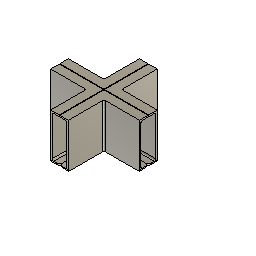
CornerProtectorForRatchetStraps (Autodesk Fusion 360 design; units mm, degrees)
Autodesk Fusion 360 part; units mm, degrees
sketch "Sketch1" plane through (0, 0, 0) normal (0, 0, 1) x (1, 0, 0)
  line L0 (0, 0) -> (0, 25)
  line L1 (0, 25) -> (1, 25)
  line L2 (1, 25) -> (1, 1)
  line L3 (1, 1) -> (25, 1)
  line L4 (25, 1) -> (25, 0)
  line L5 (25, 0) -> (0, 0)
  dimension "d1" = 1
  dimension "d2" = 25
  dimension "d3" = 25
  constraint coincident L0.start L5.end
  constraint vertical L0
  constraint perpendicular L0 L1
  constraint perpendicular L1 L2
  constraint perpendicular L2 L3
  constraint perpendicular L3 L4
  constraint horizontal L5
  constraint equal L1 L4
  measures "d1" distance of L0.end L1.end
  measures "d2" distance of L0.start L0.end
  measures "d3" distance of L4.end L0.start
extrude "Extrude2" add sketch "Sketch1" along normal blind 30
fillet "Fillet2" radius 1 2 edges at (1, 1, 15) (0, 0, 15)
ref_plane "WorkPlane1" through (12.5, 12.5, 15) normal (0, 0, 1) x (1, 0, 0)
sketch "Sketch3" plane through (0, 0, 0) normal (0, 0, 1) x (1, 0, 0)
  arc A0 (0, 1) -> (1, 0) centre (1, 1) ccw
  line L0 (0, 1) -> (0, 25)
  line L1 (0, 25) -> (1, 25)
  line L2 (1, 25) -> (1, 2)
  arc A1 (1, 2) -> (2, 1) centre (2, 2) ccw
  line L3 (2, 1) -> (25, 1)
  line L4 (25, 1) -> (25, 0)
  line L5 (25, 0) -> (1, 0)
  line L6 (0, 25) -> (-5, 25)
  line L7 (-5, 25) -> (-5, -5)
  line L8 (-5, -5) -> (25, -5)
  line L9 (25, -5) -> (25, 0)
  dimension "d16" = 5
  constraint coincident L0.end L1.start
  constraint perpendicular L0 L6
  constraint perpendicular L6 L7
  constraint perpendicular L4 L8
  constraint coincident L4.end L5.start
  constraint perpendicular L5 L9
  constraint equal L6 L9
  measures "d16" distance of L0.end L6.end
extrude "Extrude3" add sketch "Sketch3" along normal blind 1 contours A0 L0 L5 L6 L7 L8 L9
fillet "Fillet3" radius 1 3 edges at (0, 13, 1) (0.2929, 0.2929, 1) (13, 0, 1)
fillet "Fillet4" radius 2 3 edges at (-5, -5, 0.5) (25, -5, 0.5) (-5, 25, 0.5)
mirror "Mirror1" about plane through (12.5, 12.5, 15) normal (0, 0, 1) of "Extrude3", "Fillet3"
chamfer "Chamfer2" distance 0.2 distance2 0.5 2 edges at (-5, 10, 30) (10, -5, 30) measured on face at (-3, 7.3333, 30) measured on face at (-3, 7.3333, 30)
chamfer "Chamfer3" distance 1 distance2 0.2 7 edges at (-5, 10, 0) (-4.4142, -4.4142, 0) (10, -5, 0) (24.4142, -4.4142, 0) (25, -1, 0) (-1, 25, 0) (-4.4142, 24.4142, 0) measured on face at (-5, 14.3333, 0.3333) measured on face at (-4, -4.7321, 0.3333) measured on face at (5.6667, -5, 0.3333) measured on face at (23.0952, -4.9977, 0.3333) measured on face at (-3, 7.3333, 0) measured on face at (-3, 7.3333, 0) measured on face at (-3.0952, 24.9977, 0.3333)
ref_plane "WorkPlane2" through (-5, 23, 1) normal (1, 0, 0) x (0, 1, 0)
mirror "Mirror2" about plane through (-5, 23, 1) normal (1, 0, 0) of bodies 1 merged
ref_plane "WorkPlane3" through (-3, -5, 1) normal (0, 1, 0) x (-1, 0, 0)
mirror "Mirror3" about plane through (-3, -5, 1) normal (0, 1, 0) of bodies 1 merged
equation "BumpDistance = 5 mm"
named bodies: "CornerProtectorsx4"
